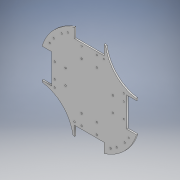
# Autodesk Inventor part: floor
Saved by Autodesk Inventor 2020 (Build 240168000, 168)
## iProperties
Created: 2024-09-07
Part Number: floor
Material: Типовые
Document SubType Name: Modeling
Designer: Ivan
Density: 1 g/cm^3
Appearance: По умолчанию
Author: Ivan
Autodesk Inventor part; units mm, degrees
ref_plane "YZ Plane" through (0, 0, 0) normal (1, 0, 0) x (0, 1, 0)
ref_plane "XZ Plane" through (0, 0, 0) normal (0, 1, 0) x (-1, 0, 0)
ref_plane "XY Plane" through (0, 0, 0) normal (0, 0, 1) x (1, 0, 0)
sketch "Эскиз2" plane through (0, 0, 0) normal (0, 0, 1) x (1, 0, 0)
  circle A0 centre (0, 0) radius 107.5
  circle A1 centre (0, 0) radius 104
  line L0 (-99.2724, 31) -> (-78.7724, 31)
  line L1 (-99.2724, -31) -> (-78.7724, -31)
  line L2 (-31, 99.2724) -> (-31, 78.7724)
  line L3 (31, 99.2724) -> (31, 78.7724)
  line L4 (99.2724, 31) -> (78.7724, 31)
  line L5 (99.2724, -31) -> (78.7724, -31)
  line L6 (31, -99.2724) -> (31, -78.7724)
  line L7 (-31, -99.2724) -> (-31, -78.7724)
  line L8 (-78.7724, -31) -> (-78.7724, 31)
  line L9 (-31, 78.7724) -> (31, 78.7724)
  line L10 (78.7724, 31) -> (78.7724, -31)
  line L11 (31, -78.7724) -> (-31, -78.7724)
  circle A2 centre (-109.0212, -109.0212) radius 75.25
  line L12 (-31, 78.7724) -> (78.7724, -31) construction
  line L13 (-73.5391, 73.5391) -> (73.5391, -73.5391) construction
  circle A3 centre (109.0212, 109.0212) radius 75.25
  point P0 (-98.0863, -34.57)
  point P1 (-34.57, -98.0863)
  point P2 (98.0863, 34.57)
  point P3 (34.57, 98.0863)
  dimension "d1" = 208
  dimension "d0" = 215
  dimension "d8" = 20.5
  dimension "d9" = 31
  dimension "d10" = 31
  dimension "d11" = 31
  dimension "d12" = 31
  dimension "d13" = 31
  dimension "d14" = 31
  dimension "d15" = 31
  dimension "d16" = 31
  dimension "d17" = 150.5
  dimension "d18" = 3.57
  dimension "d19" = 3.57
  constraints: 28 end point, 7 equal length, 4 horizontal, 4 vertical, 3 centre point, 2 coincident, 2 point on circle, 1 midpoint, 1 parallel, 1 symmetric about line, 15 other
  measures "d0" diameter of A0
  measures "d8" distance of L0.start L0.end
  measures "d9" distance from line of L0 point (0, 0)
  measures "d10" distance from line of L7 point (0, 0)
  measures "d11" distance from line of L6 point (0, 0)
  measures "d12" distance from line of L5 point (0, 0)
  measures "d13" distance from line of L4 point (0, 0)
  measures "d14" distance from line of L3 point (0, 0)
  measures "d15" distance from line of L2 A0.centre
  measures "d16" distance from line of L1 point (0, 0)
  measures "d17" diameter of A2
  measures "d18" vertical distance of L1.start A2.end
  measures "d19" horizontal distance of L7.start A2.start
extrude "Выдавливание1" add sketch "Эскиз2" along normal blind 3 contours A1 L4 L10 L5 L6 L11 L7 A2 L1 L8 L0 L2 L9 L3 A3
sketch "Эскиз3" plane through (0, 0, 0) normal (0, 0, -1) x (-1, 0, 0)
  line L0 (-78.7724, -31) -> (-78.7724, 31) projected
  line L1 (-78.7724, 16) -> (78.7724, 16) construction
  line L2 (78.7724, 31) -> (78.7724, -31) projected
  line L3 (-31, 78.7724) -> (31, 78.7724) projected
  line L4 (31, -78.7724) -> (-31, -78.7724) projected
  line L5 (-16, -78.7724) -> (-16, 78.7724) construction
  line L6 (0, 0) -> (0, 78.7724) construction
  line L7 (0, 0) -> (78.7724, 0) construction
  line L8 (-78.7724, -16) -> (78.7724, -16) construction
  line L9 (16, -78.7724) -> (16, 78.7724) construction
  circle A0 centre (-49.72, 16) radius 1.5
  circle A1 centre (-49.72, -16) radius 1.5
  circle A2 centre (-16, 49.72) radius 1.5
  circle A3 centre (16, 49.72) radius 1.5
  circle A4 centre (49.72, 16) radius 1.5
  circle A5 centre (49.72, -16) radius 1.5
  line L10 (-49.72, 49.72) -> (49.72, 49.72) construction
  line L11 (49.72, 49.72) -> (49.72, -49.72) construction
  line L12 (49.72, -49.72) -> (-49.72, -49.72) construction
  line L13 (-49.72, -49.72) -> (-49.72, 49.72) construction
  line L14 (-49.72, 49.72) -> (49.72, -49.72) construction
  circle A6 centre (-16, -49.72) radius 1.5
  circle A7 centre (16, -49.72) radius 1.5
  line L15 (-72.43, 72.43) -> (72.43, 72.43) construction
  line L16 (72.43, 72.43) -> (72.43, -72.43) construction
  line L17 (72.43, -72.43) -> (-72.43, -72.43) construction
  line L18 (-72.43, -72.43) -> (-72.43, 72.43) construction
  line L19 (-72.43, 72.43) -> (72.43, -72.43) construction
  circle A8 centre (-72.43, 16) radius 1.5
  circle A9 centre (-72.43, -16) radius 1.5
  circle A10 centre (-16, 72.43) radius 1.5
  circle A11 centre (16, 72.43) radius 1.5
  circle A12 centre (72.43, 16) radius 1.5
  circle A13 centre (72.43, -16) radius 1.5
  circle A14 centre (16, -72.43) radius 1.5
  circle A15 centre (-16, -72.43) radius 1.5
  circle A16 centre (-72.43, 31) radius 1.5
  circle A17 centre (-31, 72.43) radius 1.5
  circle A18 centre (31, -72.43) radius 1.5
  circle A19 centre (72.43, -31) radius 1.5
  line L20 (-99.2724, -31) -> (-78.7724, -31) projected
  line L21 (-31, -78.7724) -> (-31, -99.2724) projected
  arc A20 (-89.0224, -31) -> (-31, -89.0224) centre (0, 0) ccw construction
  arc A21 (89.0224, 31) -> (31, 89.0224) centre (0, 0) ccw construction
  circle A22 centre (-57.67, -74.5664) radius 1.5
  line L22 (-72.43, -72.43) -> (72.43, 72.43) construction
  circle A23 centre (-74.5664, -57.67) radius 1.5
  circle A24 centre (-44.87, -82.9015) radius 1.5
  circle A25 centre (-82.9015, -44.87) radius 1.5
  circle A26 centre (74.5664, 57.67) radius 1.5
  circle A27 centre (57.67, 74.5664) radius 1.5
  circle A28 centre (82.9015, 44.87) radius 1.5
  circle A29 centre (44.87, 82.9015) radius 1.5
  arc A30 (-98.0863, 34.57) -> (-34.57, 98.0863) centre (-109.0212, 109.0212) ccw projected
  dimension "d22" = 16
  dimension "d23" = 16
  dimension "d25" = 99.44
  dimension "d26" = 3
  dimension "d27" = 144.86
  dimension "d28" = 3
  dimension "d29" = 3
  dimension "d30" = 15
  dimension "d31" = 15
  dimension "d32" = 15
  dimension "d33" = 15
  dimension "d35" = 26.67
  dimension "d36" = 13.87
  dimension "d37" = 3
  constraints: 39 point on line, 34 end point, 30 centre point, 18 equal radius, 12 symmetric about line, 6 midpoint, 6 point on circle, 4 parallel, 4 perpendicular, 3 horizontal, 1 coincident, 1 vertical, 7 other
  measures "d22" distance from line of L1 L6.start
  measures "d23" distance from line of L5 L6.start
  measures "d25" distance of L11.end L12.end
  measures "d26" diameter of A0
  measures "d27" distance of L17.end L15.start
  measures "d28" diameter of A11
  measures "d29" diameter of A16
  measures "d30" distance of A16.centre A8.centre
  measures "d31" distance of A17.centre A10.centre
  measures "d32" distance of A13.centre A19.centre
  measures "d33" distance of A14.centre A18.centre
  measures "d35" distance from line of L21 A22.centre
  measures "d36" distance from line of L21 A24.centre
  measures "d37" diameter of A24
extrude "Выдавливание2" cut sketch "Эскиз3" against normal blind 3
